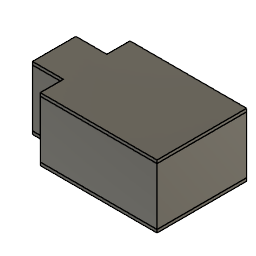
Component Box (Autodesk Fusion 360 design; units mm, degrees)
Autodesk Fusion 360 part; units mm, degrees
sketch "Sketch4" plane through (0, 0, 0) normal (0, 0, 1) x (1, 0, 0)
  line L0 (-50, 0) -> (-121.7, 0)
  line L1 (-121.7, 0) -> (-121.7, -54.2)
  line L2 (-121.7, -54.2) -> (-50, -54.2)
  line L3 (-50, -54.2) -> (-50, 0)
  line L4 (-121.7, 0) -> (-119.7, 0)
  line L5 (-121.7, 0) -> (-108.5, 0)
  line L6 (-121.7, 0) -> (-99.8, 0)
  line L7 (-121.7, 0) -> (-84.5, 0)
  line L8 (-121.7, 0) -> (-79.9, 0)
  line L9 (-121.7, 0) -> (-69.5, 0)
  line L10 (-123.7, 2) -> (-123.7, -56.2)
  line L11 (-123.7, -56.2) -> (-48, -56.2)
  line L12 (-48, -56.2) -> (-48, 2)
  line L13 (-48, 2) -> (-123.7, 2)
  dimension "d27" = 71.7
  dimension "d28" = 54.2
  dimension "d29" = 2
  dimension "d30" = 13.2
  dimension "d31" = 21.9
  dimension "d32" = 37.2
  dimension "d33" = 41.8
  dimension "d34" = 52.2
  dimension "d35" = 2
  constraint horizontal L0
  constraint vertical L1
  constraint horizontal L2
  constraint vertical L3
  constraint parallel L0 L4
  constraint perpendicular L1 L5
  constraint perpendicular L1 L6
  constraint perpendicular L1 L7
  constraint perpendicular L1 L8
  constraint perpendicular L1 L9
  measures "d27" distance of L0.start L0.end
  measures "d28" distance of L0.start L2.end
  measures "d29" distance of L0.end L4.end
  measures "d30" distance of L0.end L5.end
  measures "d31" distance of L0.end L6.end
  measures "d32" distance of L0.end L7.end
  measures "d33" distance of L0.end L8.end
  measures "d34" distance of L0.end L9.end
extrude "Extrude6" add sketch "Sketch4" along normal blind 5 contours L0 L1 L2 L3 L4 L5 L6 L7 L8 L9 makes body 1
extrude "Extrude7" add sketch "Sketch4" along normal blind 27 separate body makes body 2
move_body "Move2" bodies 1 2 to x (1, 0, 0) y (0, 1, 0) z (0, 0, 1) at (0, 0, -5)
sketch "Sketch5" plane through (0, 0, 0) normal (0, -1, 0) x (1, 0, 0)
  line L0 (-121.7, -5) -> (-50, -5)
  line L1 (-50, -5) -> (-50, 22)
  line L2 (-50, 22) -> (-121.7, 22)
  line L3 (-121.7, 22) -> (-121.7, -5)
  line L4 (-119.7, 0) -> (-108.5, 0)
  line L5 (-108.5, 0) -> (-108.5, 10)
  line L6 (-108.5, 10) -> (-119.7, 10)
  line L7 (-119.7, 10) -> (-119.7, 0)
  line L8 (-99.8, 0) -> (-84.5, 0)
  line L9 (-84.5, 0) -> (-84.5, 10)
  line L10 (-84.5, 10) -> (-99.8, 10)
  line L11 (-99.8, 10) -> (-99.8, 0)
  line L12 (-79.9, 0) -> (-69.5, 0)
  line L13 (-69.5, 0) -> (-69.5, 10)
  line L14 (-69.5, 10) -> (-79.9, 10)
  line L15 (-79.9, 10) -> (-79.9, 0)
  point P0 (-119.7, 0)
  point P1 (-108.5, 0)
  point P2 (-99.8, 0)
  point P3 (-84.5, 0)
  point P4 (-79.9, 0)
  point P5 (-69.5, 0)
  dimension "d40" = 10
  dimension "d41" = 10
  dimension "d42" = 10
  constraint horizontal L4
  constraint vertical L5
  constraint horizontal L6
  constraint vertical L7
  constraint coincident P0 L4.start
  constraint horizontal L8
  constraint vertical L9
  constraint horizontal L10
  constraint vertical L11
  constraint coincident P2 L8.start
  constraint horizontal L12
  constraint vertical L13
  constraint horizontal L14
  constraint vertical L15
  constraint coincident P4 L12.start
  measures "d40" distance of P0 L6.end
  measures "d41" distance of P2 L10.end
  measures "d42" distance of P4 L14.end
extrude "Extrude8" cut sketch "Sketch5" against normal blind 9 contours L4 L5 L6 L7 | L8 L9 L10 L11 | L12 L13 L14 L15 bodies 2
move_body "Move3" bodies 2 1 to x (1, 0, 0) y (0, 1, 0) z (0, 0, 1) at (0, 0, 5)
combine "Combine1" operation add target body 1 tool bodies 2
move_body "Move4" bodies 1 to x (1, 0, 0) y (0, 1, 0) z (0, 0, 1) at (0, -95, 0)
move_body "Move5" bodies 1 to x (1, 0, 0) y (0, 1, 0) z (0, 0, 1) at (0, 20, 0)
extrude "Extrude9" add sketch "Sketch4" along normal blind 2 separate body contours L0 L1 L2 L3 L4 L5 L6 L7 L8 L9 | L10 L11 L12 L13 makes body 3
extrude "Extrude10" add sketch "Sketch4" along normal blind 5 separate body contours L0 L1 L2 L3 L4 L5 L6 L7 L8 L9 makes body 4
combine "Combine2" operation add target body 3 tool bodies 4
move_body "Align1" bodies 1 to x (1, 0, 0) y (0, 1, 0) z (0, 0, 1) at (0, 0, 0)
move_body "Align2" bodies 1 to x (1, 0, 0) y (0, 1, 0) z (0, 0, 1) at (0, 0, 0)
move_face "OffsetFaces2" offset -7 1 faces at (-73.9, -130.5333, 27) on bodies 1
move_face "OffsetFaces3" offset -3 1 faces at (-98.4667, -92.4, 0) on bodies 1
delete_body "RemoveBody1" bodies 3
sketch "Sketch7" plane through (0, 0, 3) normal (0, 0, -1) x (1, 0, 0)
  line L0 (-123.7, 73) -> (-48, 73)
  line L1 (-48, 73) -> (-48, 131.2)
  line L2 (-48, 131.2) -> (-123.7, 131.2)
  line L3 (-123.7, 131.2) -> (-123.7, 73)
  line L4 (-48, 73) -> (-123.7, 73)
  line L5 (-123.7, 73) -> (-123.7, 131.2)
  line L6 (-123.7, 131.2) -> (-48, 131.2)
  line L7 (-48, 131.2) -> (-48, 73)
  line L8 (-121.7, 75) -> (-121.7, 129.2)
  line L9 (-121.7, 129.2) -> (-50, 129.2)
  line L10 (-50, 129.2) -> (-50, 75)
  line L11 (-50, 75) -> (-121.7, 75)
  dimension "d56" = 2
  constraint horizontal L4
  constraint vertical L5
  constraint horizontal L6
  constraint vertical L7
  constraint coincident L2.end L3.start
  constraint coincident L0.end L1.start
extrude "Extrude11" add sketch "Sketch7" along normal blind 19 bodies 1
sketch "Sketch8" plane through (0, -73, 0) normal (0, 1, 0) x (-1, 0, 0)
  line L0 (119.7, 5) -> (108.5, 5)
  line L1 (108.5, 5) -> (108.5, 15)
  line L2 (108.5, 15) -> (119.7, 15)
  line L3 (119.7, 15) -> (119.7, 5)
  line L4 (99.8, 5) -> (84.5, 5)
  line L5 (84.5, 5) -> (84.5, 15)
  line L6 (84.5, 15) -> (99.8, 15)
  line L7 (99.8, 15) -> (99.8, 5)
  line L8 (79.9, 5) -> (69.5, 5)
  line L9 (69.5, 5) -> (69.5, 15)
  line L10 (69.5, 15) -> (79.9, 15)
  line L11 (79.9, 15) -> (79.9, 5)
  line L12 (123.7, -16) -> (123.7, 20)
  line L13 (123.7, 20) -> (48, 20)
  line L14 (48, 20) -> (48, -16)
  line L15 (48, -16) -> (123.7, -16)
  line L16 (119.7, 15) -> (119.7, 5)
  line L17 (108.5, 5) -> (108.5, 15)
  line L18 (99.8, 15) -> (99.8, 5)
  line L19 (84.5, 5) -> (84.5, 15)
  line L20 (79.9, 15) -> (79.9, 5)
  line L21 (69.5, 5) -> (69.5, 15)
  line L22 (119.7, 5) -> (123.7, 5)
  line L23 (48, 3) -> (123.7, 3)
  line L24 (108.5, 5) -> (108.5, 3) construction
  line L25 (119.7, 5) -> (119.7, 3) construction
  line L26 (84.5, 5) -> (84.5, 3) construction
  line L27 (99.8, 5) -> (99.8, 3) construction
  line L28 (79.9, 5) -> (79.9, 3) construction
  line L29 (69.5, 5) -> (69.5, 3) construction
  line L30 (119.7, 3) -> (108.5, 3)
  line L31 (108.5, 3) -> (108.5, -5.4)
  line L32 (108.5, -5.4) -> (119.7, -5.4)
  line L33 (119.7, -5.4) -> (119.7, 3)
  line L34 (84.5, 3) -> (99.8, 3)
  line L35 (84.5, 3) -> (92.15, 3)
  line L36 (84.5, 3) -> (92.15, 3)
  line L37 (92.15, 3) -> (92.15, -3.7) construction
  line L38 (92.15, 3) -> (102.2, 3)
  line L39 (92.15, 3) -> (82.1, 3)
  line L40 (82.1, 3) -> (102.2, 3)
  line L41 (102.2, 3) -> (102.2, -3.7)
  line L42 (102.2, -3.7) -> (82.1, -3.7)
  line L43 (82.1, -3.7) -> (82.1, 3)
  line L44 (82.1, -3.7) -> (85.6, -3.7)
  line L45 (85.6, -3.7) -> (84.25, -3.7)
  line L46 (84.25, -3.7) -> (84.25, -0.35) construction
  line L47 (102.2, -3.7) -> (98.7, -3.7)
  line L48 (98.7, -3.7) -> (100.05, -3.7)
  line L49 (100.05, -3.7) -> (100.05, -0.35) construction
  circle A0 centre (84.25, -0.35) radius 1.4
  circle A1 centre (100.05, -0.35) radius 1.4
  line L50 (92.15, 3) -> (92.15, -0.35) construction
  line L51 (92.15, 3) -> (92.15, 2) construction
  line L52 (92.15, -3.7) -> (92.15, -2.7) construction
  line L53 (92.15, 2) -> (92.15, -2.7) construction
  line L54 (84.25, -0.35) -> (85.65, -0.35) construction
  line L55 (85.65, -0.35) -> (87.15, -0.35)
  line L56 (100.05, -0.35) -> (98.65, -0.35) construction
  line L57 (98.65, -0.35) -> (97.15, -0.35)
  line L58 (87.15, -0.35) -> (87.15, 2)
  line L59 (87.15, 2) -> (92.15, 2)
  line L60 (92.15, -2.7) -> (87.15, -2.7)
  line L61 (87.15, -2.7) -> (87.15, -0.35)
  line L62 (92.15, -2.7) -> (97.15, -2.7)
  line L63 (97.15, -2.7) -> (97.15, -0.35)
  line L64 (92.15, 2) -> (97.15, 2)
  line L65 (97.15, 2) -> (97.15, -0.35)
  line L66 (87.15, 2) -> (92.15, 2)
  dimension "d59" = 8.4
  dimension "d60" = 6.7
  dimension "d61" = 10.05
  dimension "d62" = 10.05
  dimension "d63" = 6.7
  dimension "d64" = 3.5
  dimension "d65" = 1.35
  dimension "d66" = 3.35
  dimension "d67" = 3.5
  dimension "d68" = 1.35
  dimension "d69" = 2.8
  dimension "d70" = 2.8
  dimension "d71" = 1
  dimension "d72" = 1
  dimension "d73" = 1.5
  dimension "d74" = 1.5
  constraint coincident L0.start L3.end
  constraint coincident L12 L22.end
  constraint perpendicular L12 L22
  constraint coincident L0.end L1.start
  constraint coincident L23 L24.end
  constraint perpendicular L23 L24
  constraint coincident L23 L25.end
  constraint perpendicular L23 L25
  constraint coincident L4.end L5.start
  constraint coincident L23 L26.end
  constraint perpendicular L23 L26
  constraint coincident L4.start L7.end
  constraint coincident L23 L27.end
  constraint perpendicular L23 L27
  constraint coincident L8.start L11.end
  constraint coincident L23 L28.end
  constraint perpendicular L23 L28
  constraint coincident L8.end L9.start
  constraint coincident L23 L29.end
  constraint perpendicular L23 L29
  constraint horizontal L30
  constraint vertical L31
  constraint horizontal L32
  constraint vertical L33
  constraint midpoint L34 L35.end
  constraint perpendicular L34 L37
  constraint perpendicular L37 L38
  constraint perpendicular L37 L39
  constraint horizontal L40
  constraint vertical L41
  constraint horizontal L42
  constraint vertical L43
  constraint perpendicular L43 L44
  constraint perpendicular L43 L45
  constraint perpendicular L42 L46
  constraint perpendicular L41 L47
  constraint parallel L42 L48
  constraint perpendicular L48 L49
  constraint coincident L46.end A0.centre
  constraint coincident L49.end A1.centre
  constraint midpoint L37 L50.end
  constraint perpendicular L23 L51
  constraint perpendicular L42 L52
  constraint coincident A0 L54.end
  constraint perpendicular L46 L54
  constraint perpendicular L46 L55
  constraint coincident A1 L56.end
  constraint perpendicular L49 L56
  constraint perpendicular L49 L57
  constraint perpendicular L55 L58
  constraint perpendicular L58 L60
  constraint perpendicular L55 L61
  constraint perpendicular L37 L62
  constraint perpendicular L57 L63
  constraint perpendicular L37 L64
  constraint perpendicular L57 L65
  measures "d59" distance of L25.end L32.end
  measures "d60" distance of L35.end L37.end
  measures "d61" distance of L35.end L38.end
  measures "d62" distance of L35.end L39.end
  measures "d63" distance of L39.end L42.end
  measures "d64" distance of L42.end L44.end
  measures "d65" distance of L44.end L45.end
  measures "d66" distance of L45.end L46.end
  measures "d67" distance of L41.end L47.end
  measures "d68" distance of L47.end L48.end
  measures "d69" diameter of A0
  measures "d70" diameter of A1
  measures "d71" distance of L35.end L51.end
  measures "d72" distance of L37.end L52.end
  measures "d73" distance of L54.end L55.end
  measures "d74" distance of L56.end L57.end
extrude "Extrude12" cut sketch "Sketch8" against normal blind 2.5 contours A0 | A1 | L58 L59 L60 L61 L62 L63 L64 L65 L66 bodies 1
extrude "Extrude13" cut sketch "Sketch8" against normal blind 4 contours L23 L30 L31 L32 L33 bodies 1
move_face "OffsetFaces4" offset 10 1 faces at (-112.2333, -73.6667, 15) on bodies 1
move_face "OffsetFaces5" offset -2 1 faces at (-123.7, -111.8, 8) on bodies 1
sketch "Sketch10" plane through (0, 0, 3) normal (0, 0, -1) x (1, 0, 0)
  line L0 (-121.7, 75) -> (-121.7, 129.2)
  line L1 (-121.7, 75) -> (-121.7, 102.1)
  line L2 (-121.7, 102.1) -> (-121.7, 114.2)
  line L3 (-121.7, 102.1) -> (-121.7, 90)
  line L4 (-121.7, 114.2) -> (-141.8, 114.2)
  line L5 (-141.8, 114.2) -> (-141.8, 90)
  line L6 (-141.8, 90) -> (-121.7, 90)
  line L7 (-121.7, 90) -> (-121.7, 114.2)
  line L8 (-121.7, 114.2) -> (-131.75, 114.2)
  line L9 (-121.7, 90) -> (-131.75, 90)
  line L10 (-131.75, 114.2) -> (-131.75, 113.5) construction
  line L11 (-131.75, 90) -> (-131.75, 90.7) construction
  line L12 (-131.75, 113.5) -> (-131.75, 111.7) construction
  line L13 (-131.75, 90.7) -> (-131.75, 92.5) construction
  circle A0 centre (-131.75, 111.7) radius 1.8
  circle A1 centre (-131.75, 92.5) radius 1.8
  line L14 (-119.7, 116.2) -> (-143.8, 116.2)
  line L15 (-143.8, 116.2) -> (-143.8, 88)
  line L16 (-143.8, 88) -> (-119.7, 88)
  line L17 (-119.7, 88) -> (-119.7, 116.2)
  line L18 (-123.7, 73) -> (-123.7, 131.2)
  line L19 (-123.7, 131.2) -> (-121.7, 131.2)
  line L20 (-121.7, 131.2) -> (-121.7, 116.2)
  line L21 (-121.7, 116.2) -> (-123.7, 116.2)
  line L22 (-123.7, 116.2) -> (-123.7, 131.2)
  line L23 (-123.7, 73) -> (-121.7, 73)
  line L24 (-121.7, 73) -> (-121.7, 88)
  line L25 (-121.7, 88) -> (-123.7, 88)
  line L26 (-123.7, 88) -> (-123.7, 73)
  dimension "d91" = 12.1
  dimension "d92" = 12.1
  dimension "d93" = 20.1
  dimension "d94" = 0.7
  dimension "d95" = 0.7
  dimension "d96" = 1.8
  dimension "d97" = 1.8
  dimension "d98" = 2
  constraint coincident L0.start L1.start
  constraint midpoint L0 L1.end
  constraint parallel L0 L2
  constraint parallel L0 L3
  constraint horizontal L4
  constraint vertical L5
  constraint horizontal L6
  constraint vertical L7
  constraint midpoint L4 L8.end
  constraint midpoint L6 L9.end
  constraint perpendicular L8 L10
  constraint perpendicular L9 L11
  constraint parallel L10 L12
  constraint perpendicular L6 L13
  constraint coincident L12.end A0.centre
  constraint coincident L10.end A0
  constraint coincident L13.end A1.centre
  constraint coincident L11.end A1
  constraint horizontal L19
  constraint vertical L20
  constraint horizontal L21
  constraint vertical L22
  constraint coincident L0 L20.end
  constraint coincident L14 L20.end
  constraint coincident L18.end L19.start
  constraint horizontal L23
  constraint vertical L24
  constraint horizontal L25
  constraint vertical L26
  constraint coincident L16 L24.end
  constraint coincident L1 L24.end
  constraint coincident L18.start L23.start
  measures "d91" distance of L1.end L2.end
  measures "d92" distance of L1.end L3.end
  measures "d93" distance of L2.end L4.end
  measures "d94" distance of L8.end L10.end
  measures "d95" distance of L9.end L11.end
  measures "d96" distance of L10.end L12.end
  measures "d97" distance of L11.end L13.end
extrude "Extrude14" add sketch "Sketch10" against normal up to surface (17 mm away) contours L0 L1 L16 L18 L23 L24 L25 L26 | L0 L14 L18 L19 L20 L21 L22 bodies 1
extrude "Extrude15" add sketch "Sketch10" against normal blind 2 contours L0 L1 L2 L3 L4 L6 L7 L8 L9 L18 | L4 L5 L6 L8 L9 L18 bodies 1
extrude "Extrude16" add sketch "Sketch10" along normal up to surface (19 mm away) contours L0 L1 L16 L18 L23 L24 L25 L26 | L0 L14 L18 L19 L20 L21 L22 bodies 1
extrude "Extrude17" add sketch "Sketch10" along normal up to surface (19 mm away) separate body contours L0 L1 L6 L9 L16 L18 L25 | L4 L5 L6 L8 L9 L14 L15 L16 L18 | L0 L4 L8 L14 L18 L21 makes body 5
combine "Combine3" operation add target body 1 tool bodies 5
extrude "Extrude18" add sketch "Sketch10" against normal up to surface (17 mm away) contours L0 L1 L6 L9 L16 L18 L25 | L4 L5 L6 L8 L9 L14 L15 L16 L18 | L0 L4 L8 L14 L18 L21 bodies 1
move_face "OffsetFaces6" offset 11 1 faces at (-79.9, -73.6667, 11.6667) on bodies 1
sketch "Sketch11" plane through (0, 0, 3) normal (0, 0, -1) x (1, 0, 0)
  line L0 (-121.7, 129.2) -> (-121.7, 114.2)
  line L1 (-121.7, 114.2) -> (-141.8, 114.2)
  line L2 (-141.8, 114.2) -> (-141.8, 90)
  line L3 (-141.8, 90) -> (-131.75, 90)
  line L4 (-131.75, 90) -> (-121.7, 90)
  line L5 (-121.7, 90) -> (-121.7, 75)
  line L6 (-121.7, 75) -> (-119.7, 75)
  line L7 (-119.7, 75) -> (-119.7, 73)
  line L8 (-119.7, 73) -> (-108.5, 73)
  line L9 (-108.5, 73) -> (-108.5, 75)
  line L10 (-108.5, 75) -> (-50, 75)
  line L11 (-50, 75) -> (-50, 129.2)
  line L12 (-50, 129.2) -> (-121.7, 129.2)
  circle A0 centre (-131.75, 111.7) radius 1.8
  circle A1 centre (-131.75, 92.5) radius 1.8
  line L13 (-50, 75) -> (-121.7, 75)
  line L14 (-50, 129.2) -> (-50, 75)
  line L15 (-121.7, 90) -> (-121.7, 75)
  line L16 (-121.7, 129.2) -> (-121.7, 114.2)
  line L17 (-123.7, 88) -> (-123.7, 73)
  line L18 (-123.7, 73) -> (-48, 73)
  line L19 (-48, 73) -> (-48, 131.2)
  line L20 (-48, 131.2) -> (-123.7, 131.2)
  line L21 (-123.7, 131.2) -> (-123.7, 116.2)
  line L22 (-123.7, 116.2) -> (-143.8, 116.2)
  line L23 (-143.8, 116.2) -> (-143.8, 88)
  line L24 (-143.8, 88) -> (-123.7, 88)
  line L25 (-121.7, 75) -> (-121.7, 90)
  line L26 (-121.7, 90) -> (-131.75, 90)
  line L27 (-131.75, 90) -> (-141.8, 90)
  line L28 (-141.8, 90) -> (-141.8, 114.2)
  line L29 (-141.8, 114.2) -> (-121.7, 114.2)
  line L30 (-121.7, 114.2) -> (-121.7, 129.2)
  line L31 (-121.7, 129.2) -> (-50, 129.2)
  line L32 (-50, 129.2) -> (-50, 75)
  line L33 (-50, 75) -> (-121.7, 75)
  line L34 (-50, 75) -> (-50, 80)
  line L35 (-50, 75) -> (-50, 100)
  line L36 (-50, 75) -> (-54, 75)
  line L37 (-50, 75) -> (-62.6, 75)
  line L38 (-54, 75) -> (-54, 80) construction
  line L39 (-54, 80) -> (-50, 80) construction
  line L40 (-54, 80) -> (-62.6, 80) construction
  line L41 (-54, 80) -> (-54, 100) construction
  line L42 (-54, 100) -> (-62.6, 100) construction
  line L43 (-50, 100) -> (-54, 100) construction
  line L44 (-62.6, 75) -> (-62.6, 80) construction
  line L45 (-62.6, 80) -> (-62.6, 100) construction
  line L46 (-54.5, 80.5) -> (-54.5, 99.5) construction
  line L47 (-54.5, 99.5) -> (-62.1, 99.5)
  line L48 (-62.1, 80.5) -> (-62.1, 99.5)
  line L49 (-54.5, 80.5) -> (-62.1, 80.5)
  line L50 (-62.1, 99.5) -> (-50, 99.5)
  line L51 (-50, 99.5) -> (-50, 80.5)
  line L52 (-50, 80.5) -> (-62.1, 80.5)
  line L53 (-62.1, 80.5) -> (-62.1, 99.5)
  line L54 (-50, 129.2) -> (-71.8, 129.2)
  line L55 (-121.7, 129.2) -> (-107.4, 129.2)
  line L56 (-71.8, 129.2) -> (-107.4, 129.2)
  line L57 (-107.4, 129.2) -> (-107.4, 110.8)
  line L58 (-107.4, 110.8) -> (-71.8, 110.8)
  line L59 (-71.8, 110.8) -> (-71.8, 129.2)
  dimension "d110" = 5
  dimension "d111" = 25
  dimension "d112" = 4
  dimension "d113" = 12.6
  dimension "d114" = 12.6
  dimension "d115" = -0.5
  dimension "d116" = 19
  dimension "d117" = 21.8
  dimension "d118" = 14.3
  dimension "d119" = 18.4
  constraint coincident L10.end L11.start
  constraint perpendicular L13 L34
  constraint perpendicular L13 L35
  constraint coincident L10 L36.end
  constraint perpendicular L35 L37
  constraint perpendicular L33 L38
  constraint perpendicular L41 L43
  constraint perpendicular L40 L44
  constraint perpendicular L42 L45
  constraint horizontal L50
  constraint vertical L51
  constraint horizontal L52
  constraint vertical L53
  constraint coincident L14 L51.end
  constraint coincident L11.end L12.start
  constraint perpendicular L14 L54
  constraint coincident L0.start L12.end
  constraint perpendicular L30 L55
  constraint horizontal L56
  constraint vertical L57
  constraint horizontal L58
  constraint vertical L59
  measures "d110" distance of L10.end L34.end
  measures "d111" distance of L10.end L35.end
  measures "d112" distance of L10.end L36.end
  measures "d113" distance of L10.end L37.end
  measures "d114" distance of L35.end L42.end
  measures "d116" distance of L47.end L48.start
  measures "d117" distance of L11.end L54.end
  measures "d118" distance of L0.start L55.end
  measures "d119" distance of L54.end L58.end
extrude "Extrude19" add sketch "Sketch11" along normal up to surface (19 mm away) contours L12 L31 L56 L57 L58 L59 | L11 L14 L32 L35 L47 L48 L49 L50 L51 L52 L53 bodies 1
sketch "Sketch12" plane through (0, 0, -16) normal (0, 0, -1) x (1, 0, 0)
  line L0 (-123.7, 88) -> (-123.7, 73)
  line L1 (-123.7, 73) -> (-48, 73)
  line L2 (-48, 73) -> (-48, 131.2)
  line L3 (-48, 131.2) -> (-123.7, 131.2)
  line L4 (-123.7, 131.2) -> (-123.7, 116.2)
  line L5 (-123.7, 116.2) -> (-143.8, 116.2)
  line L6 (-143.8, 116.2) -> (-143.8, 88)
  line L7 (-143.8, 88) -> (-123.7, 88)
  line L8 (-121.7, 75) -> (-121.7, 90)
  line L9 (-121.7, 90) -> (-131.75, 90)
  line L10 (-131.75, 90) -> (-141.8, 90)
  line L11 (-141.8, 90) -> (-141.8, 114.2)
  line L12 (-141.8, 114.2) -> (-121.7, 114.2)
  line L13 (-121.7, 114.2) -> (-121.7, 129.2)
  line L14 (-121.7, 129.2) -> (-107.4, 129.2)
  line L15 (-107.4, 129.2) -> (-107.4, 110.8)
  line L16 (-107.4, 110.8) -> (-71.8, 110.8)
  line L17 (-71.8, 110.8) -> (-71.8, 129.2)
  line L18 (-71.8, 129.2) -> (-50, 129.2)
  line L19 (-50, 129.2) -> (-50, 99.5)
  line L20 (-50, 99.5) -> (-62.1, 99.5)
  line L21 (-62.1, 99.5) -> (-62.1, 80.5)
  line L22 (-62.1, 80.5) -> (-50, 80.5)
  line L23 (-50, 80.5) -> (-50, 75)
  line L24 (-50, 75) -> (-121.7, 75)
  line L25 (-48, 73) -> (-48, 131.2)
  line L26 (-123.7, 116.2) -> (-123.7, 131.2)
  line L27 (-143.8, 116.2) -> (-123.7, 116.2)
  line L28 (-143.8, 88) -> (-143.8, 116.2)
  line L29 (-123.7, 88) -> (-143.8, 88)
  line L30 (-123.7, 73) -> (-123.7, 88)
  line L31 (-48, 73) -> (-123.7, 73)
  line L32 (-48, 131.2) -> (-123.7, 131.2)
  line L33 (-141.8, 90) -> (-141.8, 114.2)
  line L34 (-141.8, 114.2) -> (-121.7, 114.2)
  line L35 (-121.7, 114.2) -> (-121.7, 129.2)
  line L36 (-50, 129.2) -> (-121.7, 129.2)
  line L37 (-50, 75) -> (-50, 129.2)
  line L38 (-50, 75) -> (-121.7, 75)
  line L39 (-121.7, 75) -> (-121.7, 90)
  line L40 (-121.7, 90) -> (-141.8, 90)
  dimension "d122" = 2
extrude "Extrude20" cut sketch "Sketch7" along normal blind 2 contours L8 L9 L10 L11 bodies 1
extrude "Extrude21" cut sketch "Sketch7" against normal blind 2 contours L8 L9 L10 L11 bodies 1
extrude "Extrude22" add 2 faces at (-55.5333, -93.1667, 1) (-95.5333, -123.0667, 1) along direction (0, 0, 1) up to surface end surface through (-79.9, -75, 5) normal (0, 0, 1) offset 0 on bodies 1 bodies 1
sketch "Sketch13" plane through (0, 0, -16) normal (0, 0, -1) x (1, 0, 0)
  line L0 (-123.7, 88) -> (-123.7, 73)
  line L1 (-123.7, 73) -> (-48, 73)
  line L2 (-48, 73) -> (-48, 131.2)
  line L3 (-48, 131.2) -> (-123.7, 131.2)
  line L4 (-123.7, 131.2) -> (-123.7, 116.2)
  line L5 (-123.7, 116.2) -> (-143.8, 116.2)
  line L6 (-143.8, 116.2) -> (-143.8, 88)
  line L7 (-143.8, 88) -> (-123.7, 88)
  line L8 (-121.7, 75) -> (-121.7, 90)
  line L9 (-121.7, 90) -> (-131.75, 90)
  line L10 (-131.75, 90) -> (-141.8, 90)
  line L11 (-141.8, 90) -> (-141.8, 114.2)
  line L12 (-141.8, 114.2) -> (-121.7, 114.2)
  line L13 (-121.7, 114.2) -> (-121.7, 129.2)
  line L14 (-121.7, 129.2) -> (-107.4, 129.2)
  line L15 (-107.4, 129.2) -> (-107.4, 110.8)
  line L16 (-107.4, 110.8) -> (-71.8, 110.8)
  line L17 (-71.8, 110.8) -> (-71.8, 129.2)
  line L18 (-71.8, 129.2) -> (-50, 129.2)
  line L19 (-50, 129.2) -> (-50, 99.5)
  line L20 (-50, 99.5) -> (-62.1, 99.5)
  line L21 (-62.1, 99.5) -> (-62.1, 80.5)
  line L22 (-62.1, 80.5) -> (-50, 80.5)
  line L23 (-50, 80.5) -> (-50, 75)
  line L24 (-50, 75) -> (-121.7, 75)
  line L25 (-107.4, 110.8) -> (-107.4, 129.2)
  line L26 (-71.8, 110.8) -> (-107.4, 110.8)
  line L27 (-121.7, 75) -> (-116.7, 75)
  line L28 (-116.7, 75) -> (-116.7, 84)
  line L29 (-107.4, 110.8) -> (-107.4, 75)
  line L30 (-121.7, 90) -> (-116.7, 90)
  line L31 (-116.7, 90) -> (-116.7, 84)
  line L32 (-116.7, 84) -> (-121.7, 84)
  line L33 (-121.7, 84) -> (-121.7, 90)
  line L34 (-116.7, 84) -> (-107.4, 84)
  line L35 (-107.4, 84) -> (-107.4, 90)
  line L36 (-107.4, 90) -> (-116.7, 90)
  line L37 (-116.7, 90) -> (-116.7, 84)
  dimension "d129" = 5
  dimension "d130" = 9
  constraint coincident L8.start L24.end
  constraint perpendicular L8 L27
  constraint perpendicular L27 L28
  constraint coincident L15.end L16.start
  constraint coincident L24 L29.end
  constraint perpendicular L24 L29
  constraint horizontal L30
  constraint vertical L31
  constraint horizontal L32
  constraint vertical L33
  constraint coincident L8.end L9.start
  constraint horizontal L34
  constraint vertical L35
  constraint horizontal L36
  constraint vertical L37
  constraint coincident L29 L35.end
  measures "d129" distance of L8.start L27.end
  measures "d130" distance of L27.end L28.end
extrude "Extrude23" add sketch "Sketch13" against normal up to surface (21 mm away) contours L8 L30 L31 L32 L33 L37 | L29 L31 L34 L35 L36 L37 bodies 1
move_face "OffsetFaces7" offset 1 1 faces at (-95.5333, -123.0667, -16) on bodies 1
sketch "Sketch14" plane through (0, 0, -17) normal (0, 0, -1) x (1, 0, 0)
  line L0 (-123.7, 88) -> (-123.7, 73)
  line L1 (-123.7, 73) -> (-48, 73)
  line L2 (-48, 73) -> (-48, 131.2)
  line L3 (-48, 131.2) -> (-123.7, 131.2)
  line L4 (-123.7, 131.2) -> (-123.7, 116.2)
  line L5 (-123.7, 116.2) -> (-143.8, 116.2)
  line L6 (-143.8, 116.2) -> (-143.8, 88)
  line L7 (-143.8, 88) -> (-123.7, 88)
  line L8 (-121.7, 90) -> (-131.75, 90)
  line L9 (-131.75, 90) -> (-141.8, 90)
  line L10 (-141.8, 90) -> (-141.8, 114.2)
  line L11 (-141.8, 114.2) -> (-121.7, 114.2)
  line L12 (-121.7, 114.2) -> (-121.7, 129.2)
  line L13 (-121.7, 129.2) -> (-107.4, 129.2)
  line L14 (-107.4, 129.2) -> (-107.4, 110.8)
  line L15 (-107.4, 110.8) -> (-71.8, 110.8)
  line L16 (-71.8, 110.8) -> (-71.8, 129.2)
  line L17 (-71.8, 129.2) -> (-50, 129.2)
  line L18 (-50, 129.2) -> (-50, 99.5)
  line L19 (-50, 99.5) -> (-62.1, 99.5)
  line L20 (-62.1, 99.5) -> (-62.1, 80.5)
  line L21 (-62.1, 80.5) -> (-50, 80.5)
  line L22 (-50, 80.5) -> (-50, 75)
  line L23 (-50, 75) -> (-121.7, 75)
  line L24 (-121.7, 75) -> (-121.7, 84)
  line L25 (-121.7, 84) -> (-107.4, 84)
  line L26 (-107.4, 84) -> (-107.4, 90)
  line L27 (-107.4, 90) -> (-121.7, 90)
extrude "Extrude24" add sketch "Sketch14" against normal blind 2 separate body contours L8 L9 L10 L11 L12 L13 L14 L15 L16 L17 L18 L19 L20 L21 L22 L23 L24 L25 L26 L27 makes body 6
extrude "Extrude25" add sketch "Sketch14" along normal blind 2 separate body contours L0 L1 L2 L3 L4 L5 L6 L7 | L8 L9 L10 L11 L12 L13 L14 L15 L16 L17 L18 L19 L20 L21 L22 L23 L24 L25 L26 L27 makes body 7
combine "Combine4" operation add target body 6 tool bodies 7
move_face "OffsetFaces8" offset -0.15 20 faces at (-107.4, -86, -16.3333) (-116.9333, -84, -16.3333) (-121.7, -78, -16.3333) (-112.1667, -90, -16.3333) (-125.05, -90, -16.3333) (-135.1, -90, -16.3333) (-141.8, -98.0667, -15.6667) (-73.9, -75, -16.3333) (-54.0333, -99.5, -16.3333) (-121.7, -119.2, -16.3333) (-135.1, -114.2, -16.3333) (-116.9333, -129.2, -16.3333) (-95.5333, -110.8, -16.3333) (-71.8, -116.9333, -16.3333) (-64.5333, -129.2, -16.3333) (-58.0667, -80.5, -16.3333) (-107.4, -123.0667, -16.3333) (-50, -119.3, -16.3333) (-62.1, -93.1667, -15.6667) (-50, -78.6667, -16.3333) on bodies 6
sketch "Sketch15" plane through (0, 0, 20) normal (0, 0, 1) x (-1, 0, 0)
  line L0 (121.7, 90) -> (121.7, 75)
  line L1 (121.7, 75) -> (50, 75)
  line L2 (50, 75) -> (50, 129.2)
  line L3 (50, 129.2) -> (121.7, 129.2)
  line L4 (121.7, 129.2) -> (121.7, 114.2)
  line L5 (121.7, 114.2) -> (141.8, 114.2)
  line L6 (141.8, 114.2) -> (141.8, 90)
  line L7 (141.8, 90) -> (131.75, 90)
  line L8 (131.75, 90) -> (121.7, 90)
  line L9 (123.7, 88) -> (143.8, 88)
  line L10 (143.8, 88) -> (143.8, 116.2)
  line L11 (143.8, 116.2) -> (123.7, 116.2)
  line L12 (123.7, 116.2) -> (123.7, 131.2)
  line L13 (123.7, 131.2) -> (48, 131.2)
  line L14 (48, 131.2) -> (48, 73)
  line L15 (48, 73) -> (123.7, 73)
  line L16 (123.7, 73) -> (123.7, 88)
extrude "Extrude26" add sketch "Sketch15" against normal blind 2 separate body contours L0 L1 L2 L3 L4 L5 L6 L7 L8 makes body 8
extrude "Extrude27" add sketch "Sketch15" along normal blind 2 separate body contours L0 L1 L2 L3 L4 L5 L6 L7 L8 | L9 L10 L11 L12 L13 L14 L15 L16 makes body 9
combine "Combine5" operation add target body 8 tool bodies 9
move_face "OffsetFaces9" offset -0.15 9 faces at (-73.9, -129.2, 19.3333) (-121.7, -124.2, 19.3333) (-128.4, -114.2, 19.3333) (-141.8, -106.1333, 18.6667) (-121.7, -85, 19.3333) (-128.4, -90, 19.3333) (-138.45, -90, 19.3333) (-97.8, -75, 19.3333) (-50, -93.0667, 19.3333) on bodies 8
sketch "Sketch9" plane through (0, 0, 3) normal (0, 0, -1) x (1, 0, 0)
  line L0 (-122, 129) -> (-122, 75)
  line L1 (-122, 129) -> (-122, 102)
  line L2 (-122, 102) -> (-142.1, 102) construction
  line L3 (-142.1, 102) -> (-142.1, 114.1)
  line L4 (-142.1, 102) -> (-142.1, 89.9)
  line L5 (-142.1, 114.1) -> (-121.9998, 114.1)
  line L6 (-142.1, 89.9) -> (-122, 89.9)
  line L7 (-144.1, 116.1) -> (-121.9998, 116.1)
  line L8 (-144.1, 102) -> (-144.1, 116.1)
  line L9 (-144.1, 102) -> (-144.1, 87.9)
  line L10 (-144.1, 87.9) -> (-122, 87.9)
  line L11 (-142.1, 102) -> (-142.1, 103.8)
  line L12 (-142.1, 102) -> (-142.1, 100.2)
  line L13 (-142.1, 114.1) -> (-132.0499, 114.1)
  line L14 (-132.0499, 114.1) -> (-132.0499, 113.4)
  line L15 (-132.0499, 113.4) -> (-132.0499, 111.6)
  circle A0 centre (-132.0499, 111.6) radius 1.8
  line L16 (-142.1, 89.9) -> (-132.05, 89.9)
  line L17 (-132.05, 89.9) -> (-132.05, 90.6)
  line L18 (-132.05, 90.6) -> (-132.05, 92.4)
  circle A1 centre (-132.05, 92.4) radius 1.8
  line L19 (-123.7, 73) -> (-123.7, 131.2)
  line L20 (-119.7, 73) -> (-123.7, 73)
  line L21 (-123.7, 131.2) -> (-48, 131.2)
  line L22 (-48, 73) -> (-123.7, 73)
  line L23 (-48, 131.2) -> (-48, 73)
  line L24 (-121.7, 75) -> (-121.7, 129.2)
  line L25 (-122, 75) -> (-122, 73)
  line L26 (-122, 129) -> (-122, 131.2)
  dimension "d81" = 20.1
  dimension "d82" = 12.1
  dimension "d83" = 12.1
  dimension "d84" = -2
  dimension "d85" = 1.8
  dimension "d86" = 1.8
  dimension "d87" = 0.7
  dimension "d88" = 1.8
  dimension "d89" = 0.7
  dimension "d90" = 1.8
  constraint vertical L0
  constraint midpoint L0 L1.end
  constraint perpendicular L1 L2
  constraint perpendicular L2 L3
  constraint perpendicular L2 L4
  constraint horizontal L5
  constraint coincident L0 L6.end
  constraint perpendicular L0 L6
  constraint perpendicular L2 L11
  constraint perpendicular L2 L12
  constraint midpoint L5 L13.end
  constraint perpendicular L5 L14
  constraint perpendicular L5 L15
  constraint coincident L15.end A0.centre
  constraint coincident L14.end A0
  constraint midpoint L6 L16.end
  constraint perpendicular L16 L17
  constraint parallel L17 L18
  constraint coincident L18.end A1.centre
  constraint coincident L17.end A1
  constraint coincident L22 L25.end
  constraint coincident L21 L26.end
  constraint perpendicular L21 L26
  measures "d81" distance of L1.end L2.end
  measures "d82" distance of L2.end L3.end
  measures "d83" distance of L2.end L4.end
  measures "d85" distance of L2.end L11.end
  measures "d86" distance of L2.end L12.end
  measures "d87" distance of L13.end L14.end
  measures "d88" distance of L14.end L15.end
  measures "d89" distance of L16.end L17.end
  measures "d90" distance of L17.end L18.end
move_face "OffsetFaces1" [suppressed]
named bodies: "Box", "Bottom Lid", "Top Lid"
